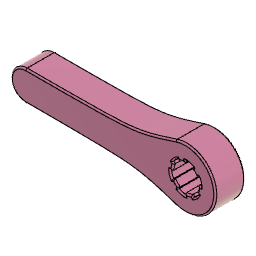
Spezialschluessel (Autodesk Fusion 360 design; units mm, degrees)
Autodesk Fusion 360 part; units mm, degrees
sketch "Sketch1" plane through (0, 0, 0) normal (0, 1, 0) x (1, 0, 0)
  circle A0 centre (0, 0) radius 15.25
  circle A1 centre (-160, 0) radius 15
  line L0 (0, 0) -> (0, -15.25)
  circle A2 centre (0, 0) radius 13
  line L1 (0, 0) -> (7.4901, -13.2838)
  line L2 (0, 0) -> (15.2492, -0.1553)
  line L3 (0, 0) -> (13.2069, -7.625)
  line L4 (0, 0) -> (7.7591, 13.1286)
  line L5 (0, 0) -> (13.2069, 7.625)
  line L6 (0, 0) -> (-7.4901, 13.2838)
  line L7 (0, 0) -> (0, 15.25)
  line L8 (0, 0) -> (-15.2492, 0.1553)
  line L9 (0, 0) -> (-13.2069, 7.625)
  line L10 (0, 0) -> (-7.7591, -13.1286)
  line L11 (0, 0) -> (-13.2069, -7.625)
  circle A3 centre (0, 0) radius 30
  circle A4 centre (-160, 0) radius 1.5
  spline S0 degree 2 poles (-160, 15) (-50, 15) (-9.4591, 28.4697) knots 0 0 0 15.194627 15.194627 15.194627 weights 1 3 1
  spline S1 degree 2 poles (-160, -15) (-50, -15) (-9.4591, -28.4697) knots 0 0 0 15.194627 15.194627 15.194627 weights 1 3 1
  line L12 (-150, -7.5) -> (-35, -7.5)
  arc A5 (-35, -7.5) -> (-35, 7.5) centre (-35, 0) ccw
  line L13 (-35, 7.5) -> (-150, 7.5)
  arc A6 (-150, 7.5) -> (-150, -7.5) centre (-150, 0) ccw
  line L14 (-150, 0) -> (-35, 0) construction
  dimension "d1" = 30
  dimension "d3" = 30.5
  dimension "d6" = 29.417
  dimension "d8" = 360
  dimension "d11" = 26
  dimension "d25" = 60
  dimension "d38" = 160
  dimension "d39" = 15
  dimension "d40" = 15
  dimension "d41" = 50
  dimension "d48" = 7.5
  constraint coincident A0.centre L0.start
  constraint horizontal A0.centre A1.centre
  constraint coincident A0 L0.end
  constraint vertical L0
  constraint coincident A0 L1.end
  constraint concentric A1 A4
  constraint coincident A3 S0.end
  constraint coincident A1 S0.start
  constraint tangent A3 S0
  constraint tangent A1 S0
  constraint coincident A3 S1.end
  constraint coincident A1 S1.start
  constraint tangent A3 S1
  constraint tangent A1 S1
  constraint tangent L12 A5
  constraint tangent A5 L13
  constraint parallel L12 L13
  constraint tangent L13 A6
  constraint tangent L12 A6
  constraint horizontal L14
  measures "d1" diameter of A1
  measures "d3" diameter of A0
  measures "d6" angle of L0 L1
  measures "d11" diameter of A2
  measures "d25" diameter of A3
  measures "d38" distance of A0.centre A1.centre
  measures "d48" radius of A5
extrude "Extrude1" add sketch "Sketch1" along normal blind 30 contours A0 A2 L2 L5 | A0 A2 L4 L7 | A0 A2 L1 L3 | A0 A2 L6 L9 | A0 L0 A2 L10 | A0 A2 L8 L11 | A1 L12 L13 A6 | A1 A3 S0 A5 L13 | A1 A3 S1 L12 A5 | A1 A3 L12 A5 L13 | A1 L12 L13 A6 | A3 A5 | A3 A5 | A4
fillet "Fillet2" radius 1.5 56 edges at (0, 0, 14.125) (-7.1867, 0, 12.1601) (-10.8381, 0, 10.7283) (-12.574, 0, 3.3007) (-3.4285, 0, 12.5397) (-14.7101, 0, -4.0219) (-14.1243, 0, -0.1438) (-12.2326, 0, 7.0625) (-9.1455, 0, -9.2391) (-12.2326, 0, -7.0625) (-6.9376, 0, -12.3039) (-3.872, 0, -14.7503) (3.4285, 0, -12.5397) (0, 0, -14.125) (10.8381, 0, -10.7283) (7.1867, 0, -12.1601) (12.574, 0, -3.3007) (12.2326, 0, -7.0625) (14.7101, 0, 4.0219) (14.1243, 0, 0.1438) (9.1455, 0, 9.2391) (12.2326, 0, 7.0625) (3.872, 0, 14.7503) (6.9376, 0, 12.3039) (6.9376, 30, 12.3039) (3.872, 30, 14.7503) (12.2326, 30, 7.0625) (9.1455, 30, 9.2391) (14.1243, 30, 0.1438) (14.7101, 30, 4.0219) (12.2326, 30, -7.0625) (12.574, 30, -3.3007) (7.1867, 30, -12.1601) (10.8381, 30, -10.7283) (0, 30, -14.125) (3.4285, 30, -12.5397) (-6.9376, 30, -12.3039) (-3.872, 30, -14.7503) (-12.2326, 30, -7.0625) (-9.1455, 30, -9.2391) (-14.1243, 30, -0.1438) (-14.7101, 30, -4.0219) (-12.2326, 30, 7.0625) (-3.4285, 30, 12.5397) (-12.574, 30, 3.3007) (-10.8381, 30, 10.7283) (-7.1867, 30, 12.1601) (0, 30, 14.125) (-58.6824, 30, 16.6837) (30, 30, 0) (-58.6824, 30, -16.6837) (-175, 30, 0) (-58.6824, 0, -16.6837) (30, 0, 0) (-58.6824, 0, 16.6837) (-175, 0, 0)
extrude "Extrude5" cut sketch "Sketch1" along normal blind 20 and the other way blind -10 contours A1 A3 L12 A5 L13 | A1 L12 L13 A6 | A3 A5 picked at (-148.8745, -1.9026) picked at (-29.1395, 0.1721)
equation "d6 = ( ( 365 / 12 ) * 1 deg ) - 1 deg"
equation "d40 = d39"
